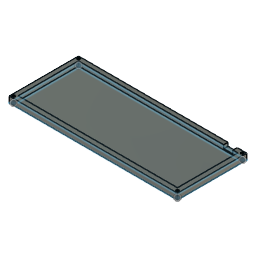
KeyboardBottom (Autodesk Fusion 360 design; units mm, degrees)
part number: 2026-01-12-19-14-13-415
Autodesk Fusion 360 part; units mm, degrees
sketch "Sketch1" plane through (0, 0, 0) normal (0, 0, 1) x (1, 0, 0)
  line L0 (0, 250) -> (351, 250)
  line L1 (351, 250) -> (351, 383)
  line L2 (351, 383) -> (0, 383)
  line L3 (0, 383) -> (0, 250)
  line L4 (-9.5, 392.5) -> (361.5, 392.5)
  line L5 (361.5, 392.5) -> (361.5, 239.5)
  line L6 (361.5, 239.5) -> (-9.5, 239.5)
  line L7 (-9.5, 239.5) -> (-9.5, 392.5)
  circle A0 centre (-4.5, 244.5) radius 1.7
  circle A1 centre (356.5, 244.5) radius 1.7
  circle A2 centre (-4.5, 387.5) radius 1.7
  circle A3 centre (356.5, 387.5) radius 1.7
  circle A4 centre (-4.5, 387.5) radius 3
  circle A5 centre (356.5, 244.5) radius 3
  circle A6 centre (-4.5, 244.5) radius 3
  circle A7 centre (356.5, 387.5) radius 3
  dimension "d1" = 351
  dimension "d2" = 133
  dimension "d3" = 371
  dimension "d4" = 153
  dimension "d5" = 9.5
  dimension "d10" = 9.5
  dimension "d11" = 3.4
  dimension "d12" = 5
  dimension "d13" = 5
  dimension "d14" = 3.4
  dimension "d15" = 5
  dimension "d16" = 5
  dimension "d17" = 3.4
  dimension "d18" = 5
  dimension "d19" = 5
  dimension "d21" = 5
  dimension "d22" = 5
  dimension "d23" = 6
  dimension "d24" = 6
  dimension "d25" = 6
  dimension "d26" = 6
  constraint horizontal L0
  constraint vertical L1
  constraint horizontal L2
  constraint vertical L3
  constraint horizontal L4
  constraint vertical L5
  constraint horizontal L6
  constraint vertical L7
  constraint coincident A2.centre A4.centre
  constraint coincident A0.centre A6.centre
  constraint coincident A1.centre A5.centre
  constraint coincident A3.centre A7.centre
  measures "d1" distance of L0.start L0.end
  measures "d2" distance of L0.start L2.end
  measures "d3" distance of L4.start L4.end
  measures "d4" distance of L4.start L6.end
  measures "d5" distance of L3 L7
  measures "d10" distance of L2 L4
  measures "d11" diameter of A0
  measures "d12" distance of L6 A0.centre
  measures "d13" distance of L7 A0.centre
  measures "d14" diameter of A1
  measures "d15" distance of L6 A1.centre
  measures "d16" distance of L5 A1.centre
  measures "d17" diameter of A2
  measures "d18" distance of L4 A2.centre
  measures "d19" distance of L7 A2.centre
  measures "d21" distance of L4 A3.centre
  measures "d22" distance of L5 A3.centre
  measures "d23" diameter of A4
  measures "d24" diameter of A5
  measures "d25" diameter of A6
  measures "d26" diameter of A7
extrude "Extrude1" add sketch "Sketch1" along normal blind 10 from surface at 3.1 contours A4 | A5 | A6 | A7 makes body 1 at (-1.5928, 245.2403, 9.7667) makes body 2 at (357.3125, 247.3879, 9.7667) makes body 3 at (-7.0599, 389.0643, 9.7667) makes body 4 at (355.1314, 384.8304, 6.4333)
extrude "Extrude2" add sketch "Sketch1" along normal blind 13 contours L4 L5 L6 L7 bodies 1 2 3 4
extrude "Extrude3" add sketch "Sketch1" along normal blind 3 contours L0 L1 L2 L3 bodies 1
sketch "Sketch2" plane through (0, 0, 13) normal (0, 0, 1) x (-1, 0, 0)
  line L0 (0, -250) -> (0, -383)
  line L1 (0, -383) -> (-351, -383)
  line L2 (-351, -383) -> (-351, -250)
  line L3 (-351, -250) -> (0, -250)
  circle A0 centre (-356.5, -244.5) radius 3
  circle A1 centre (4.5, -244.5) radius 3
  circle A2 centre (4.5, -387.5) radius 3
  circle A3 centre (-356.5, -387.5) radius 3
  line L4 (9.5, -239.5) -> (-361.5, -239.5)
  line L5 (-361.5, -239.5) -> (-361.5, -392.5)
  line L6 (-361.5, -392.5) -> (9.5, -392.5)
  line L7 (9.5, -392.5) -> (9.5, -239.5)
sketch "Sketch3" plane through (0, 0, 13) normal (0, 0, 1) x (-1, 0, 0)
  line L0 (2440, -1230) -> (2470, -1230)
  line L1 (2470, -1230) -> (2470, -1260)
  line L2 (2470, -1260) -> (2440, -1260)
  line L3 (2440, -1260) -> (2440, -1230)
  constraint horizontal L0
  constraint vertical L1
  constraint horizontal L2
  constraint vertical L3
sketch "Sketch4" plane through (0, 0, 0) normal (1, 0, 0) x (0, 1, 0)
sketch "Sketch5" plane through (0, 0, 0) normal (0, 0, 1) x (1, 0, 0)
extrude "Extrude4" cut sketch "Sketch3" against normal blind 7.5 bodies 1
sketch "Sketch6" plane through (0, 0, 13) normal (0, 0, 1) x (-1, 0, 0)
  line L0 (-320, -400) -> (-340, -400)
  line L1 (-340, -400) -> (-340, -380)
  line L2 (-340, -380) -> (-320, -380)
  line L3 (-320, -380) -> (-320, -400)
  constraint horizontal L0
  constraint vertical L1
  constraint horizontal L2
  constraint vertical L3
extrude "Extrude5" cut sketch "Sketch6" against normal blind 7.5 bodies 1
